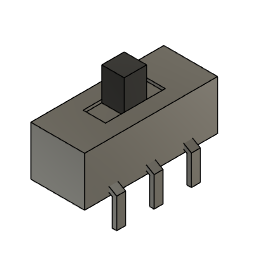
01, Test Housing v1.2 (Autodesk Fusion 360 archive; units mm, degrees)
design "Switch"
Autodesk Fusion 360 part; units mm, degrees
note: some values were not read from the file. Chosen so that the rebuilt part matches the saved one: which bodies a step acts on; a side. Set by a fixed rule: which sketch regions a step uses.
sketch "Sketch1" plane through (0, 0, 0) normal (0, 0, 1) x (1, 0, 0)
  line L0 (1.8, -4.45) -> (-1.8, -4.45)
  line L1 (-1.8, -4.45) -> (-1.8, 4.45)
  line L2 (-1.8, 4.45) -> (1.8, 4.45)
  line L3 (1.8, 4.45) -> (1.8, -4.45)
  line L4 (1.8, -4.45) -> (-1.8, 4.45) construction
  line L5 (-1.8, -4.45) -> (1.8, 4.45) construction
  line L6 (-0.75, 2) -> (0.75, 2)
  line L7 (0.75, 2) -> (0.75, -2)
  line L8 (0.75, -2) -> (-0.75, -2)
  line L9 (-0.75, -2) -> (-0.75, 2)
  line L10 (-0.75, 2) -> (0.75, -2) construction
  line L11 (0.75, 2) -> (-0.75, -2) construction
  line L12 (0.75, -0.75) -> (-0.75, -0.75)
  line L13 (-0.75, -0.75) -> (-0.75, 0.75)
  line L14 (-0.75, 0.75) -> (0.75, 0.75)
  line L15 (0.75, 0.75) -> (0.75, -0.75)
  line L16 (0.75, -0.75) -> (-0.75, 0.75) construction
  line L17 (-0.75, -0.75) -> (0.75, 0.75) construction
  dimension "d1" = 3.6
  dimension "d2" = 8.9
  dimension "d3" = 4
  dimension "d4" = 1.5
  dimension "d5" = 1.5
  constraint horizontal L0
  constraint perpendicular L0 L1
  constraint parallel L0 L2
  constraint parallel L1 L3
  constraint coincident L4 origin
  constraint coincident L5 origin
  constraint horizontal L6
  constraint perpendicular L6 L7
  constraint parallel L6 L8
  constraint parallel L7 L9
  constraint coincident L10 origin
  constraint coincident L11 origin
  constraint horizontal L12
  constraint perpendicular L12 L13
  constraint parallel L12 L14
  constraint parallel L13 L15
  constraint coincident L16 origin
  constraint coincident L17 origin
  constraint coincident L7 L12.start
  measures "d1" distance of L1.end L2.end
  measures "d2" distance of L0.end L1.end
  measures "d3" distance of L6.end L7.end
  measures "d4" distance of L7.end L8.end
  measures "d5" distance of L12.start L14.end
extrude "Extrude1" add sketch "Sketch1" against normal blind 3.3 contours L0 L1 L2 L3 | L6 L7 L9 L14 | L7 L9 L12 L13 L14 L15 | L7 L8 L9 L12 makes body 1
extrude "Extrude2" cut sketch "Sketch1" against normal blind 0.2 contours L6 L7 L9 L14 | L7 L9 L12 L13 L14 L15 | L7 L8 L9 L12 bodies 1
extrude "Extrude3" add sketch "Sketch1" along normal blind 2 and the other way up to surface (0.2 mm away) separate body contours L7 L9 L12 L13 L14 L15 makes body 2
sketch "Sketch2" plane through (0, 0, 0) normal (0, 1, 0) x (1, 0, 0)
  line L0 (1.5, 2.6) -> (2.3, 3.0619)
  line L1 (2.3, 3.0619) -> (2.3, 5.0619)
  line L2 (1.8, 0) -> (1.8, 3.3) construction
  dimension "d14" = 1.5
  dimension "d15" = 2.6
  dimension "d16" = 60
  dimension "d17" = 2
  dimension "d18" = 0.5
  constraint vertical L1
  measures "d14" horizontal distance of origin L0.start
  measures "d15" vertical distance of origin L0.start
  measures "d16" angle of L0 L2
  measures "d17" vertical distance of L0.end L1.end
  measures "d18" distance of L1 L2
extrude "Extrude4" add sketch "Sketch2" along normal mid plane 0.6 thin wall 0.3 on the left separate body open curves L0 L1 makes body 3
pattern_linear "R-Pattern1" count 3 spacing 2.5 along (0, 1, 0) both ways of bodies 3 makes body 4 at (2.3, 2.4, -3.7285) makes body 5 at (2.3, -2.6, -3.7285)

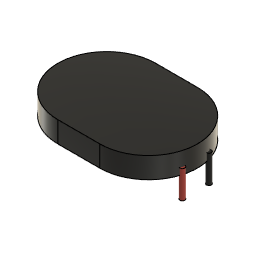
design "Echo Atom, Speaker Only"
Autodesk Fusion 360 part; units mm, degrees
sketch "Layout Sketch" plane through (0, 0, 0) normal (0, 0, 1) x (1, 0, 0)
  line L0 (-3, -7) -> (3, -7)
  arc A0 (3, -7) -> (3, 7) centre (3, 0) ccw
  line L1 (3, 7) -> (-3, 7)
  arc A1 (-3, 7) -> (-3, -7) centre (-3, 0) ccw
  line L2 (-3, 0) -> (3, 0) construction
  circle A2 centre (0, 0) radius 5.9
  circle A3 centre (9.7372, 1.9) radius 0.35
  circle A4 centre (9.7372, -1.9) radius 0.35
  dimension "d1" = 14
  dimension "d2" = 20
  dimension "d5" = 11.8
  dimension "d6" = 3.8
  dimension "d7" = 0.7
  constraint tangent L0 A0
  constraint tangent A0 L1
  constraint parallel L0 L1
  constraint tangent L1 A1
  constraint tangent L0 A1
  constraint horizontal L2
  constraint coincident A2.centre origin
  constraint midpoint L2 A2.centre
  constraint coincident A0 A3.centre
  constraint symmetric L2 A3 A4
  measures "d1" distance of L0 L1
  measures "d5" diameter of A2
  measures "d6" distance of A3.centre A4.centre
  measures "d7" diameter of A4
extrude "Extrude1" add sketch "Layout Sketch" against normal blind 3 contours L0 A0 L1 A1 A3 A4 | A0 A4 | A0 A3 | A2 picked at (9.6223, -1.8765) picked at (9.6223, 1.8765) makes body 1
extrude "Extrude2" add sketch "Layout Sketch" against normal blind 4 contours A2 bodies 1
extrude "Extrude3" add sketch "Layout Sketch" along normal blind -3 and the other way blind -1 from surface at -3 separate body contours A0 A4 | A0 A4 | A0 A3 | A0 A3 makes body 2 at (9.7459, -1.5501, -4.6667) makes body 3 at (9.7459, 2.2499, -4.6667)

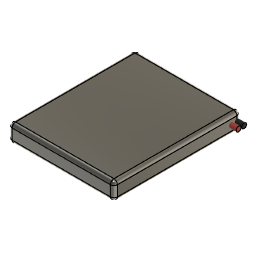
design "Battery"
Autodesk Fusion 360 part; units mm, degrees
sketch "Sketch1" plane through (0, 0, 0) normal (0, 0, 1) x (1, 0, 0)
  line L0 (0, 0) -> (30, 0)
  line L1 (30, 0) -> (30, 36)
  line L2 (30, 36) -> (0, 36)
  line L3 (0, 36) -> (0, 0)
  dimension "d1" = 36
  dimension "d2" = 30
  constraint horizontal L0
  constraint vertical L1
  constraint horizontal L2
  constraint vertical L3
  constraint coincident L0.start L3.end
  measures "d1" distance of L0.start L2.end
  measures "d2" distance of L0.start L0.end
extrude "Extrude1" add sketch "Sketch1" along normal blind 5 makes body 1
sketch "Sketch2" plane through (30, 0, 0) normal (1, 0, 0) x (0, 1, 0)
  line L0 (0, 0) -> (36, 0) construction
  line L1 (36, 0) -> (36, 5) construction
  line L2 (36, 5) -> (0, 5) construction
  line L3 (0, 5) -> (0, 0) construction
  circle A0 centre (35.1, 2.5) radius 0.7
  circle A1 centre (33.5, 2.5) radius 0.7
  line L4 (36, 2.5) -> (33.5, 2.5) construction
  dimension "d5" = 1.4
  dimension "d6" = 0.2
  dimension "d13" = 0.2
  constraint midpoint L1 L4.start
  constraint coincident A1.centre L4.end
  constraint coincident A0.centre L4
  constraint horizontal L4
  constraint equal A0 A1
  measures "d5" diameter of A0
  measures "d6" distance of L1 A0
  measures "d13" distance of A0 A1
extrude "Extrude2" add sketch "Sketch2" along normal blind 2 and the other way blind 1 separate body makes body 2 at (31.3333, 34.7807, 1.8771) makes body 3 at (31.3333, 33.1807, 1.8771)
fillet "Fillet1" radius 1 4 faces at (10, 0, 1.6667) (30, 12, 1.6667) (0, 24, 1.6667) (20, 36, 1.6667) on bodies 1
equation "d13 = d6"

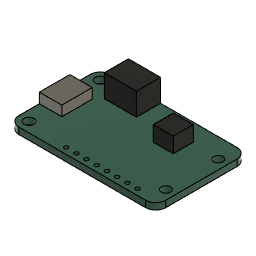
design "Power Management IC Development Tools Rechargeable 5V Lipo USB Boost"
Autodesk Fusion 360 part; units mm, degrees
sketch "Sketch1" plane through (0, 0, 0) normal (0, 0, 1) x (1, 0, 0)
  line L0 (0, -11.4) -> (36.6, -11.4)
  line L1 (36.6, -11.4) -> (36.6, 11.4)
  line L2 (36.6, 11.4) -> (0, 11.4)
  line L3 (0, 11.4) -> (0, -11.4)
  line L4 (0, 0) -> (36.6, 0)
  line L5 (5.6, -3.8) -> (0, -3.8)
  line L6 (0, -3.8) -> (0, 3.8)
  line L7 (0, 3.8) -> (5.6, 3.8)
  line L8 (5.6, 3.8) -> (5.6, -3.8)
  line L9 (5.6, -3.8) -> (0, 3.8) construction
  line L10 (0, -3.8) -> (5.6, 3.8) construction
  circle A0 centre (2.5, -8.9) radius 1.25
  circle A1 centre (34.3, -6.55) radius 1.15
  line L11 (7, 11.4) -> (15, 11.4)
  line L12 (15, 11.4) -> (15, 5.4)
  line L13 (15, 5.4) -> (7, 5.4)
  line L14 (7, 5.4) -> (7, 11.4)
  line L15 (7, 11.4) -> (15, 5.4) construction
  line L16 (15, 11.4) -> (7, 5.4) construction
  circle A2 centre (2.5, 8.9) radius 1.25
  circle A3 centre (34.3, 6.55) radius 1.15
  circle A4 centre (12.8, -9.9) radius 0.5
  circle A5 centre (15.34, -9.9) radius 0.5
  circle A6 centre (17.88, -9.9) radius 0.5
  circle A7 centre (20.42, -9.9) radius 0.5
  circle A8 centre (22.96, -9.9) radius 0.5
  circle A9 centre (25.5, -9.9) radius 0.5
  circle A10 centre (28.04, -9.9) radius 0.5
  circle A11 centre (30.58, -9.9) radius 0.5
  line L17 (27.5, 2.1) -> (22.5, 2.1)
  line L18 (22.5, 2.1) -> (22.5, 7.1)
  line L19 (22.5, 7.1) -> (27.5, 7.1)
  line L20 (27.5, 7.1) -> (27.5, 2.1)
  point P0 (2.8, 0)
  point P1 (11, 8.4)
  dimension "d1" = 36.6
  dimension "d2" = 22.8
  dimension "d3" = 5.6
  dimension "d4" = 7.6
  dimension "d5" = 8
  dimension "d6" = 7
  dimension "d7" = 6
  dimension "d8" = 17.8
  dimension "d9" = 2.5
  dimension "d10" = 2.5
  dimension "d11" = 2.3
  dimension "d12" = 13.1
  dimension "d16" = 34.3
  dimension "d17" = 1
  dimension "d18" = 12.8
  dimension "d19" = 1.5
  dimension "d22" = 2.54
  dimension "d23" = 0
  dimension "d30" = 22.5
  dimension "d31" = 4.3
  dimension "d32" = 5
  dimension "d33" = 5
  constraint horizontal L0
  constraint vertical L1
  constraint horizontal L2
  constraint vertical L3
  constraint midpoint L4.start L3
  constraint coincident L4.start origin
  constraint midpoint L1 L4.end
  constraint horizontal L5
  constraint perpendicular L5 L6
  constraint parallel L5 L7
  constraint parallel L6 L8
  constraint coincident L9 P0
  constraint coincident L10 P0
  constraint coincident L4 P0
  constraint coincident L3 L5.end
  constraint horizontal L11
  constraint perpendicular L11 L12
  constraint parallel L11 L13
  constraint parallel L12 L14
  constraint coincident L15 P1
  constraint coincident L16 P1
  constraint coincident L2 L11.start
  constraint symmetric L4 A0 A2
  constraint symmetric L4 A1 A3
  constraint horizontal L17
  constraint vertical L18
  constraint horizontal L19
  constraint vertical L20
  measures "d1" distance of L0.start L0.end
  measures "d2" distance of L0.start L2.end
  measures "d3" distance of L5.start L5.end
  measures "d4" distance of L5.start L7.end
  measures "d5" distance of L12.end L13.end
  measures "d6" distance of L3 L14
  measures "d7" distance of L11.end L12.end
  measures "d8" distance of A0.centre A2.centre
  measures "d9" diameter of A0
  measures "d10" distance of L3 A0.centre
  measures "d11" diameter of A1
  measures "d12" distance of A1.centre A3.centre
  measures "d16" distance of L3 A1.centre
  measures "d17" diameter of A4
  measures "d18" distance of L3 A4.centre
  measures "d19" distance of L0 A4.centre
  measures "d30" distance of L3 L18
  measures "d31" distance of L2 L19
  measures "d32" distance of L18.end L19.end
  measures "d33" distance of L17.end L18.end
extrude "Extrude1" add sketch "Sketch1" against normal blind 1.6 contours L0 L1 L3 L4 L5 L8 | L3 L4 L5 L6 L8 | L1 L2 L3 L4 L7 L8 L12 L13 L14 | L3 L4 L6 L7 L8 | L2 L11 L12 L13 L14 | L17 L18 L19 L20 makes body 1
extrude "Extrude2" add sketch "Sketch1" along normal blind 2.5 separate body contours L3 L4 L5 L6 L8 | L3 L4 L6 L7 L8 makes body 2
extrude "Extrude3" add sketch "Sketch1" along normal blind 5.6 separate body contours L2 L11 L12 L13 L14 makes body 3
extrude "Extrude4" add sketch "Sketch1" along normal blind 3.8 separate body contours L17 L18 L19 L20 makes body 4
fillet "Fillet1" radius 2.5 4 edges at (0, -11.4, -0.8) (0, 11.4, -0.8) (36.6, -11.4, -0.8) (36.6, 11.4, -0.8) on bodies 1
